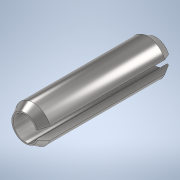
# Autodesk Inventor part: Part003.ElasticPin
Saved by Autodesk Inventor 2022.2 (Build 262287010, 287A)
## iProperties
Created: 2022-11-28
Part Number: Part003.ElasticPin
Material: Steel, Carbon
Document SubType Name: Modeling
Designer: User
Mass: 0.908365 g
Surface Area: 3.51701 cm^2
Volume: 0.115715 cm^3
Density: 7.85 g/cm^3
Appearance: Semi-Polished
Author: User
Autodesk Inventor part; units mm, degrees
ref_plane "YZ Plane" through (0, 0, 0) normal (1, 0, 0) x (0, 1, 0)
ref_plane "XZ Plane" through (0, 0, 0) normal (0, 1, 0) x (-1, 0, 0)
ref_plane "XY Plane" through (0, 0, 0) normal (0, 0, 1) x (1, 0, 0)
sketch "Sketch1" plane through (0, 0, 0) normal (0, 0, 1) x (1, 0, 0)
  arc A0 (2.0651, 0.7586) -> (2.0651, -0.7586) centre (0, 0) ccw
  arc A1 (1.3611, 0.5) -> (1.3611, -0.5) centre (0, 0) ccw
  line L0 (0, 0) -> (1.3611, 0.5) construction
  line L1 (0, 0) -> (1.3611, -0.5) construction
  arc A2 (2.0651, -0.7586) -> (2.0651, 0.7586) centre (0, 0) ccw construction
  arc A3 (1.3611, -0.5) -> (1.3611, 0.5) centre (0, 0) ccw construction
  line L2 (1.3611, 0.5) -> (2.0651, 0.7586)
  line L3 (1.3611, -0.5) -> (2.0651, -0.7586)
  point P0 (2.2, 0)
  dimension "d0" = 4.4
  dimension "d1" = 2.9
  dimension "d2" = 1
  constraints: 9 point on circle, 8 end point, 4 centre point, 2 coincident, 2 collinear, 1 horizontal alignment
  measures "d0" diameter of A0
  measures "d1" diameter of A1
  measures "d2" distance of L1.end L0.end
extrude "Extrusion1" add sketch "Sketch1" along normal blind 16
chamfer "Chamfer1" distance 1 angle 30 2 edges at (-2.2, 0, 16) (-2.2, 0, 0) measured on face at (0.8773, -2.0175, 10.6667)
body "Solid1"
